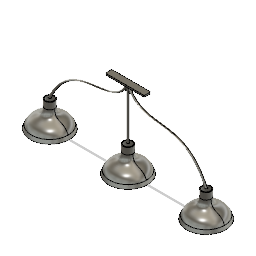
gd1 v0 (Autodesk Fusion 360 design; units mm, degrees)
Autodesk Fusion 360 part; units mm, degrees
sketch "Sketch1" plane through (0, 0, 0) normal (0, 0, 1) x (1, 0, 0)
  line L0 (-609.6, 0) -> (609.6, 0)
  line L1 (-609.6, 0) -> (-609.6, -203.2)
  line L2 (0, 0) -> (0, -203.2)
  line L3 (609.6, 0) -> (609.6, -109.1528)
  line L4 (-609.6, -203.2) -> (-457.2, -203.2)
  line L5 (-457.2, -203.2) -> (-466.8348, -176.7287)
  line L6 (-571.5, 0) -> (-571.5, -50.8)
  spline S0 degree 5 poles (-571.5, -50.8) (-571.5, -60.9196) (-569.8119, -78.7532) (-562.2206, -98.2945) (-543.76, -112.6796) (-514.1506, -123.0894) (-491.2529, -135.6067) (-477.3724, -152.5006) (-470.0286, -167.9536) (-466.8348, -176.7287) knots 0 0 0 0 0 0 0.2 0.4 0.6 0.8 1 1 1 1 1 1
  line L7 (-475.5221, -152.8605) -> (-458.1474, -200.5969)
  line L8 (-571.5, -25.4) -> (-571.5, -76.2)
  dimension "d1" = 1219.2
  dimension "d2" = 203.2
  dimension "d3" = 70
  dimension "d4" = 152.4
  dimension "d5" = 50.8
  dimension "d6" = 38.1
  dimension "d7" = 50.8
  dimension "d8" = 50.8
  constraint horizontal L0
  constraint midpoint L2.start L0
  constraint perpendicular L0 L1
  constraint coincident L2.start origin
  constraint perpendicular L0 L2
  constraint perpendicular L0 L3
  constraint equal L1 L2
  constraint perpendicular L1 L4
  constraint coincident L0 L6.start
  constraint perpendicular L0 L6
  constraint midpoint L5.end L7
  constraint midpoint L6.end L8
  constraint vertical L8
  constraint collinear L5 L7
  measures "d1" distance of L0.start L0.end
  measures "d2" distance of L0.start L1.end
  measures "d3" angle of L4 L5
  measures "d4" distance of L1.end L4.end
  measures "d5" distance of L7.start L7.end
  measures "d6" distance of L1 L6
  measures "d7" distance of L6.start L6.end
  measures "d8" distance of L8.start L8.end
revolve "Revolve1" add sketch "Sketch1" angle 360 about axis through (-609.6, 0, 0) along (0, -1, 0) makes body 1
pattern_linear "R-Pattern1" count 3 spacing 609.6 along (1, 0, 0) of bodies 1 makes body 2 at (-78.2703, -125.8843, 59.2874) makes body 3 at (626.6505, -125.8843, 96.6981)
sketch "Sketch2" plane through (0, 0, 0) normal (0, 0, 1) x (1, 0, 0)
  line L0 (-152.4, 412.75) -> (152.4, 412.75)
  line L1 (152.4, 412.75) -> (152.4, 400.05)
  line L2 (152.4, 400.05) -> (-152.4, 400.05)
  line L3 (-152.4, 400.05) -> (-152.4, 412.75)
  line L4 (-152.4, 412.75) -> (152.4, 400.05) construction
  line L5 (152.4, 412.75) -> (-152.4, 400.05) construction
  point P0 (0, 406.4)
  dimension "d14" = 12.7
  dimension "d15" = 304.8
  dimension "d16" = 406.4
  constraint perpendicular L0 L1
  constraint parallel L0 L2
  constraint parallel L1 L3
  constraint horizontal L0
  constraint coincident L4 P0
  constraint coincident L5 P0
  constraint vertical origin P0
  measures "d14" distance of L0.end L1.end
  measures "d15" distance of L1.end L2.end
  measures "d16" distance of origin P0
extrude "Extrude1" add sketch "Sketch2" along normal mid plane 50.8 separate body makes body 4
fillet "Fillet1" radius 6.35 4 edges at (152.4, 406.4, 25.4) (152.4, 406.4, -25.4) (-152.4, 406.4, -25.4) (-152.4, 406.4, 25.4) on bodies 4
shell "Shell1" thickness 6.35 removed faces 6 at (-599.1917, 0, 2.0302) at (-617.5469, -203.2, -50.1746) at (16.6088, 0, 10.3042) at (60.5323, -203.2, -25.4109) at (610.9714, 0, -7.0283) at (655.0987, -203.2, -55.5981) on bodies 1 2 3
ref_plane "WorkPlane1" through (0, 406.4, 0) normal (0, 0, 1) x (1, 0, 0)
sketch "Sketch3" plane through (0, 406.4, 0) normal (0, 0, 1) x (1, 0, 0)
  spline S0 degree 5 poles (0, 0) (0, -16.256) (0, -48.768) (0, -97.536) (0, -162.56) (0, -243.84) (0, -308.864) (0, -357.632) (0, -390.144) (0, -406.4) knots 0 0 0 0 0 0 0.2 0.4 0.6 0.8 1 1 1 1 1 1
  spline S1 degree 5 poles (0, 0) (3.3771, -9.2092) (10.749, -26.8632) (23.6603, -51.0506) (44.6087, -78.681) (77.0687, -105.503) (115.6629, -124.9301) (159.8922, -137.8726) (208.6331, -146.2287) (260.2978, -152.6261) (313.0994, -159.9993) (365.2731, -171.224) (415.2867, -188.7681) (462.1175, -214.2162) (505.217, -248.3442) (544.342, -291.4286) (572.4275, -333.0355) (591.7039, -368.1922) (603.7661, -393.3735) (609.6, -406.4) knots 0 0 0 0 0 0 0.066667 0.133333 0.2 0.266667 0.333333 0.4 0.466667 0.533333 0.6 0.666667 0.733333 0.8 0.866667 0.933333 1 1 1 1 1 1
  line L0 (0, -406.4) -> (0, 101.6) construction
  spline S2 degree 5 poles (0, 0) (-3.3771, -9.2092) (-10.749, -26.8632) (-23.6603, -51.0506) (-44.6087, -78.681) (-77.0687, -105.503) (-115.6629, -124.9301) (-159.8922, -137.8726) (-208.6331, -146.2287) (-260.2978, -152.6261) (-313.0994, -159.9993) (-365.2731, -171.224) (-415.2867, -188.7681) (-462.1175, -214.2162) (-505.217, -248.3442) (-544.342, -291.4286) (-572.4275, -333.0355) (-591.7039, -368.1922) (-603.7661, -393.3735) (-609.6, -406.4) knots 0 0 0 0 0 0 0.066667 0.133333 0.2 0.266667 0.333333 0.4 0.466667 0.533333 0.6 0.666667 0.733333 0.8 0.866667 0.933333 1 1 1 1 1 1
  line L1 (-31.6554, 86.3241) -> (31.6554, -86.3241)
  line L2 (568.344, -314.2797) -> (650.8559, -498.5203)
  line L3 (31.6554, 86.3241) -> (-31.6554, -86.3241)
  line L4 (-568.344, -314.2797) -> (-650.8559, -498.5203)
  point P0 (127, -127)
  point P1 (381, -177.8)
  point P2 (-127, -127)
  point P3 (-381, -177.8)
  constraint coincident S0.start S1.start
  constraint vertical L0
  constraint midpoint S0.start L1
  constraint midpoint S1.end L2
  constraint symmetric S0.start L0 S1.start
  constraint symmetric P0 L0 P2
  constraint symmetric P1 L0 P3
  constraint symmetric S1.end L0 S2.end
  constraint symmetric L0 L1.start L3.start
  constraint symmetric L0 L1.end L3.end
  constraint symmetric L0 L2.start L4.start
  constraint symmetric L0 L2.end L4.end
sketch "Sketch4" plane through (0, 412.75, 0) normal (0, 1, 0) x (-1, 0, 0)
  arc A0 (152.4, 19.05) -> (146.05, 25.4) centre (146.05, 19.05) ccw
  line L0 (146.05, 25.4) -> (-146.05, 25.4)
  arc A1 (-146.05, 25.4) -> (-152.4, 19.05) centre (-146.05, 19.05) ccw
  line L1 (-152.4, 19.05) -> (-152.4, -19.05)
  arc A2 (-152.4, -19.05) -> (-146.05, -25.4) centre (-146.05, -19.05) ccw
  line L2 (-146.05, -25.4) -> (146.05, -25.4)
  arc A3 (146.05, -25.4) -> (152.4, -19.05) centre (146.05, -19.05) ccw
  line L3 (152.4, -19.05) -> (152.4, 19.05)
  circle A4 centre (0, 0) radius 10
  dimension "d21" = 20
  constraint coincident A4.centre origin
  measures "d21" diameter of A4
sweep "Sweep1" add kept parallel profiles "Sketch4" path "Sketch3" along S2 section 1 contours A4 bodies 4
sweep "Sweep2" add kept parallel profiles "Sketch4" path "Sketch3" along S0 section 1 contours A4 bodies 4
sweep "Sweep3" add kept parallel profiles "Sketch4" path "Sketch3" along S1 section 1 contours A4 bodies 4
sketch "Sketch6" plane through (0, 406.4, 0) normal (0, 0, 1) x (1, 0, 0)
  line L0 (-35.56, -55.88) -> (33.02, -55.88)
  line L1 (33.02, -55.88) -> (22.86, -40.64)
  line L2 (22.86, -40.64) -> (-22.86, -40.64)
  line L3 (-22.86, -40.64) -> (-35.56, -55.88)
  constraint horizontal L0
  constraint parallel L0 L2
extrude "Extrude2" add sketch "Sketch6" along normal mid plane 7.62 bodies 4
